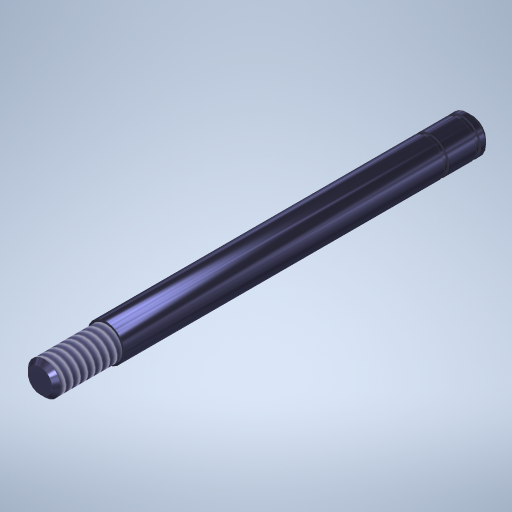
# Autodesk Inventor part: Shock Shaft
Saved by Autodesk Inventor 2023.1 (Build 271208000, 208)
## iProperties
Created: 2019-11-29
Part Number: Shock Shaft
Material: Generic
Document SubType Name: Modeling
Designer: Jopa
Density: 1 g/cm^3
Appearance: Default
Author: Jopa
Autodesk Inventor part; units mm, degrees
ref_plane "YZ Plane" through (0, 0, 0) normal (1, 0, 0) x (0, 1, 0)
sketch "Sketch1" plane through (0, 0, 0) normal (0, 0, 1) x (1, 0, 0)
  circle A0 centre (0, 0) radius 1.5875
  dimension "d0" = 3.175
  constraints: 1 centre point, 1 coincident
  measures "d0" diameter of A0
extrude "Extrusion1" add sketch "Sketch1" along normal mid plane 31.75
sketch "Sketch2" plane through (0, 0, 15.875) normal (0, 0, 1) x (1, 0, 0)
  circle A0 centre (0, 0) radius 1.4224
  dimension "d3" = 2.8448
  constraints: 1 centre point, 1 coincident
  measures "d3" diameter of A0
extrude "Extrusion2" add sketch "Sketch2" along normal blind 5.715
ref_plane "Work Plane1" through (0, 0, -15.0622) normal (0, 0, -1) x (-1, 0, 0)
sketch "Sketch3" plane through (0, 0, -15.0622) normal (0, 0, -1) x (-1, 0, 0)
  circle A0 centre (0, 0) radius 1.4224 projected
  circle A1 centre (0, 0) radius 1.5875 projected
extrude "Extrusion3" cut sketch "Sketch3" against normal blind 0.381
ref_plane "Work Plane2" through (0, 0, -12.3) normal (0, 0, -1) x (-1, 0, 0)
sketch "Sketch4" plane through (0, 0, -12.3) normal (0, 0, -1) x (-1, 0, 0)
  circle A0 centre (0, 0) radius 1.4224 projected
  circle A1 centre (0, 0) radius 1.5875 projected
extrude "Extrusion4" cut sketch "Sketch4" against normal blind 0.381
chamfer "Chamfer1" distance 0.381 angle 45 2 edges at (-1.5875, 0, -15.875) (-1.4224, 0, 21.59)
thread "Thread1" size "4-40 UNC" class "2A" standard "ANSI Unified Screw Threads" full length
body "Solid1"
